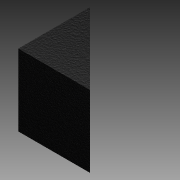
# Autodesk Inventor part: Winkel 45x45 mit Nutführung Nut 10
Saved by Autodesk Inventor 2012 SP1 (Build 160190100, 190)
## iProperties
Created: 2013-05-07
Part Number: Winkel 45x45 mit Nutführung Nut 10
Material: Default
Document SubType Name: Modeling
Designer: vogel
Density: 1 g/cm^3
Author: vogel
Autodesk Inventor part; units mm, degrees
ref_plane "YZ Plane" through (0, 0, 0) normal (1, 0, 0) x (0, 1, 0)
ref_plane "XZ Plane" through (0, 0, 0) normal (0, 1, 0) x (-1, 0, 0)
ref_plane "XY Plane" through (0, 0, 0) normal (0, 0, 1) x (1, 0, 0)
sketch "Skizze1" plane through (0, 0, 0) normal (0, 0, 1) x (1, 0, 0)
  line L0 (0, 0) -> (0, 45)
  line L1 (0, 45) -> (45, 0)
  line L2 (45, 0) -> (0, 0)
  dimension "d0" = 45
  dimension "d1" = 45
  constraints: 6 end point, 1 perpendicular, 1 vertical
  measures "d0" angle of L0 L1
  measures "d1" distance of L0.start L0.end
extrude "Extrusion1" add sketch "Skizze1" along normal blind 45
